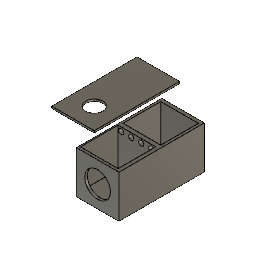
boite projet v02 (Autodesk Fusion 360 design; units mm, degrees)
Autodesk Fusion 360 part; units mm, degrees
sketch "Esquisse1" plane through (0, 0, 0) normal (1, 0, 0) x (0, 1, 0)
  line L0 (50, 25) -> (-50, 25)
  line L1 (-50, 25) -> (-50, -25)
  line L2 (-50, -25) -> (50, -25)
  line L3 (50, -25) -> (50, 25)
  line L4 (50, 25) -> (-50, -25) construction
  line L5 (-50, 25) -> (50, -25) construction
  line L6 (-45.5279, 22.7639) -> (-2.2988, 22.7639)
  line L7 (-2.2988, 22.7639) -> (-2.2988, -22.3105)
  line L8 (-2.2988, -22.3105) -> (-45.5279, -22.3105)
  line L9 (-45.5279, -22.3105) -> (-45.5279, 22.7639)
  line L10 (45.5279, -22.7639) -> (2.2988, -22.7639)
  line L11 (45.5279, 22.3105) -> (45.5279, -22.7639)
  line L12 (2.2988, 22.3105) -> (45.5279, 22.3105)
  line L13 (2.2988, -22.7639) -> (2.2988, 22.3105)
  dimension "d5" = 100
  dimension "d6" = 50
  dimension "d7" = 5
  dimension "d9" = 360
  constraint horizontal L0
  constraint perpendicular L0 L1
  constraint parallel L0 L2
  constraint parallel L1 L3
  constraint coincident L4 origin
  constraint coincident L5 origin
  constraint horizontal L6
  constraint vertical L7
  constraint horizontal L8
  constraint vertical L9
  constraint coincident L5 L6.start
  measures "d5" distance of L1.end L2.end
  measures "d6" distance of L0.end L1.end
  measures "d7" distance of L0.end L6.start
extrude "Extrusion1" add sketch "Esquisse1" along normal blind 50 contours L0 L1 L2 L3 | L6 L7 L8 L9 | L10 L11 L12 L13 makes body 1
sketch "Esquisse2" plane through (0, 0, 25) normal (0, 0, 1) x (-1, 0, 0)
  line L0 (0, -50) -> (0, 50)
  line L1 (0, 50) -> (-50, 50)
  line L2 (-50, 50) -> (-50, -50)
  line L3 (-50, -50) -> (0, -50)
  line L4 (-2.8897, -45.9196) -> (-47, -45.9196)
  line L5 (-47, -45.9196) -> (-47, -1.8093)
  line L6 (-47, -1.8093) -> (-2.8897, -1.8093)
  line L7 (-2.8897, -1.8093) -> (-2.8897, -45.9196)
  line L8 (-1.8093, 47) -> (-1.8093, 2.8897)
  line L9 (-1.8093, 2.8897) -> (-45.9196, 2.8897)
  line L10 (-45.9196, 2.8897) -> (-45.9196, 47)
  line L11 (-45.9196, 47) -> (-1.8093, 47)
  dimension "d12" = 5
  dimension "d13" = 3
  dimension "d15" = 90
  constraint horizontal L4
  constraint vertical L5
  constraint horizontal L6
  constraint vertical L7
  constraint equal L5 L6
  measures "d12" distance of L0.start L4.start
  measures "d13" distance of L2 L5
extrude "Extrusion2" cut sketch "Esquisse2" against normal blind 45 contours L4 L5 L6 L7 | L8 L9 L10 L11 bodies 1
sketch "Esquisse3" plane through (0, -50, 0) normal (0, -1, 0) x (1, 0, 0)
  line L0 (0, 25) -> (0, -25)
  line L1 (0, -25) -> (50, -25)
  line L2 (50, -25) -> (50, 25)
  line L3 (50, 25) -> (0, 25)
  circle A0 centre (25, 0) radius 15
  dimension "d20" = 30
  dimension "d21" = 25
  dimension "d22" = 25
  measures "d20" diameter of A0
  measures "d21" vertical distance of L0.start A0.centre
  measures "d22" distance of origin A0.centre
extrude "Extrusion3" cut sketch "Esquisse3" against normal blind 5 contours A0 bodies 1
sketch "Esquisse4" plane through (0, -2.8897, 0) normal (0, -1, 0) x (1, 0, 0)
  line L0 (45.9196, 25) -> (1.8093, 25)
  line L1 (1.8093, 25) -> (1.8093, -20)
  line L2 (1.8093, -20) -> (45.9196, -20)
  line L3 (45.9196, -20) -> (45.9196, 25)
  circle A0 centre (5.5216, 20.3119) radius 3
  circle A1 centre (17.1883, 20.3119) radius 3
  circle A2 centre (28.855, 20.3119) radius 3
  circle A3 centre (40.5216, 20.3119) radius 3
  point P0 (17.1883, 20.3119)
  point P1 (28.855, 20.3119)
  point P2 (40.5216, 20.3119)
  dimension "d25" = 6
  dimension "d28" = 35
  dimension "d29" = 0
  dimension "d30" = 6
  dimension "d31" = 6
  dimension "d32" = 6
  constraint coincident P0 A1.centre
  constraint coincident P1 A2.centre
  constraint coincident P2 A3.centre
  measures "d25" diameter of A0
  measures "d30" diameter of A1
  measures "d31" diameter of A2
  measures "d32" diameter of A3
extrude "Extrusion4" cut sketch "Esquisse4" against normal blind 5 contours A0 | A1 | A2 | A3 bodies 1
sketch "Esquisse5" plane through (0, 50, 0) normal (0, 1, 0) x (-1, 0, 0)
  line L0 (0, -25) -> (0, 25)
  line L1 (0, 25) -> (-50, 25)
  line L2 (-50, 25) -> (-50, -25)
  line L3 (-50, -25) -> (0, -25)
  circle A0 centre (-24.4949, -5) radius 3
  dimension "d35" = 6
  dimension "d36" = 30
  dimension "d37" = 25
  measures "d35" diameter of A0
  measures "d36" vertical distance of L1.end A0.centre
  measures "d37" distance of origin A0.centre
extrude "Extrusion5" cut sketch "Esquisse5" against normal blind 5 contours A0 bodies 1
sketch "Esquisse6" plane through (0, 0, 0) normal (0, 0, 1) x (1, 0, 0)
  line L0 (-28.9446, 0) -> (-78.9446, 0)
  line L1 (-78.9446, 0) -> (-78.9446, 100)
  line L2 (-78.9446, 100) -> (-28.9446, 100)
  line L3 (-28.9446, 100) -> (-28.9446, 0)
  dimension "d40" = 100
  dimension "d41" = 50
  constraint horizontal L0
  constraint vertical L1
  constraint horizontal L2
  constraint vertical L3
  measures "d40" distance of L0.start L2.end
  measures "d41" distance of L0.start L0.end
sketch "Esquisse7" plane through (0, 0, 0) normal (0, 0, 1) x (1, 0, 0)
extrude "Extrusion6" add sketch "Esquisse6" along normal blind 2.5 separate body makes body 2
sketch "Esquisse8" plane through (0, 0, 2.5) normal (0, 0, 1) x (-1, 0, 0)
  line L0 (28.9446, -100) -> (78.9446, -100)
  line L1 (78.9446, -100) -> (78.9446, 0)
  line L2 (78.9446, 0) -> (28.9446, 0)
  line L3 (28.9446, 0) -> (28.9446, -100)
  circle A0 centre (53.9446, -25) radius 10
  dimension "d44" = 25
  dimension "d45" = 20
  dimension "d46" = 25
  measures "d44" distance of L2 A0.centre
  measures "d45" diameter of A0
  measures "d46" distance of L1 A0.centre
extrude "Extrusion7" cut sketch "Esquisse8" against normal blind 2.5 contours A0 bodies 2
equation "largeur = 50 mm"
equation "longueur = 100 mm"
equation "hauteur = 50 mm"
equation "trou = 45 mm"
equation "d5 = longueur"
equation "d6 = largeur"
equation "d10 = hauteur"
equation "d16 = -trou"
equation "cercle = 30 mm"
equation "petitcercle = 6 mm"
equation "d20 = cercle"
equation "d25 = petitcercle"
equation "d30 = petitcercle"
equation "d31 = petitcercle"
equation "d32 = petitcercle"
equation "d35 = petitcercle"
equation "d40 = longueur"
equation "d41 = largeur"
equation "d46 = largeur / 2"
